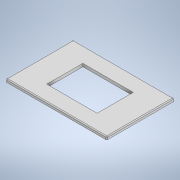
# Autodesk Inventor part: señales_tapa_x10
Saved by Autodesk Inventor 2022 (Build 260153000, 153)
## iProperties
Created: 2023-06-20
Part Number: señales_tapa_x10
Material: Generic
Document SubType Name: Modeling
Designer: Asus
Density: 1 g/cm^3
Appearance: Default
Author: Asus
Autodesk Inventor part; units mm, degrees
ref_plane "YZ Plane" through (0, 0, 0) normal (1, 0, 0) x (0, 1, 0)
ref_plane "XZ Plane" through (0, 0, 0) normal (0, 1, 0) x (-1, 0, 0)
ref_plane "XY Plane" through (0, 0, 0) normal (0, 0, 1) x (1, 0, 0)
sketch "Sketch1" plane through (0, 0, 0) normal (0, 1, 0) x (-1, 0, 0)
  line L0 (-600, 400) -> (600, 400)
  line L1 (600, 400) -> (600, -400)
  line L2 (600, -400) -> (-600, -400)
  line L3 (-600, -400) -> (-600, 400)
  line L4 (-600, 400) -> (600, -400) construction
  line L5 (600, 400) -> (-600, -400) construction
  point P0 (0, 0)
  dimension "d0" = 1200
  dimension "d1" = 800
  constraints: 12 end point, 2 midpoint, 2 parallel, 1 horizontal, 1 perpendicular
  measures "d0" distance of L1.end L2.end
  measures "d1" distance of L0.end L1.end
extrude "Extrusion1" add sketch "Sketch1" along normal blind 35
sketch "Sketch2" plane through (0, 35, 0) normal (0, 1, 0) x (1, 0, 0)
  line L0 (-300, -215) -> (300, -215)
  line L1 (300, -215) -> (300, 215)
  line L2 (300, 215) -> (-300, 215)
  line L3 (-300, 215) -> (-300, -215)
  line L4 (-300, -215) -> (300, 215) construction
  line L5 (300, -215) -> (-300, 215) construction
  point P0 (0, 0)
  dimension "d8" = 430
  dimension "d9" = 600
  constraints: 12 end point, 2 midpoint, 2 parallel, 1 horizontal, 1 perpendicular
  measures "d8" distance of L2.end L0.start
  measures "d9" distance of L1.end L2.end
extrude "Extrusion2" cut sketch "Sketch2" against normal blind 35
fillet "Fillet2" radius 10 4 edges at (0, 35, 400) (-600, 35, 0) (0, 35, -400) (600, 35, 0)
fillet "Fillet3" radius 10 8 edges at (597.0711, 32.0711, 397.0711) (600, 12.5, 400) (597.0711, 32.0711, -397.0711) (600, 12.5, -400) (-597.0711, 32.0711, 397.0711) (-600, 12.5, 400) (-597.0711, 32.0711, -397.0711) (-600, 12.5, -400)
body "Solid1"
